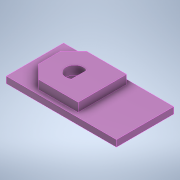
# Autodesk Inventor part: AngleSensor
Saved by Autodesk Inventor 2022 (Build 260153000, 153)
## iProperties
Created: 2021-12-29
Part Number: AngleSensor
Material: Genérico
Document SubType Name: Modeling
Designer: JK
Density: 1 g/cm^3
Appearance: Suave - Púrpura
Author: JK
Autodesk Inventor part; units mm, degrees
ref_plane "YZ Plane" through (0, 0, 0) normal (1, 0, 0) x (0, 1, 0)
ref_plane "XZ Plane" through (0, 0, 0) normal (0, 1, 0) x (-1, 0, 0)
ref_plane "XY Plane" through (0, 0, 0) normal (0, 0, 1) x (1, 0, 0)
sketch "Boceto1" plane through (0, 0, 0) normal (0, 1, 0) x (-1, 0, 0)
  line L0 (-12.5, 6.5) -> (12.5, 6.5)
  line L1 (12.5, 6.5) -> (12.5, -6.5)
  line L2 (12.5, -6.5) -> (-12.5, -6.5)
  line L3 (-12.5, -6.5) -> (-12.5, 6.5)
  line L4 (-12.5, 6.5) -> (12.5, -6.5) construction
  line L5 (12.5, 6.5) -> (-12.5, -6.5) construction
  point P0 (0, 0)
  dimension "d0" = 13
  dimension "d1" = 25
  constraints: 12 end point, 2 midpoint, 2 parallel, 1 horizontal, 1 perpendicular
  measures "d0" distance of L0.end L1.end
  measures "d1" distance of L1.end L2.end
extrude "Extrusión1" add sketch "Boceto1" along normal blind 1.5
sketch "Boceto2" plane through (0, 1.5, 0) normal (0, 1, 0) x (1, 0, 0)
  circle A0 centre (-3.5, 0) radius 2.75
  line L0 (-12.5, 6.5) -> (-12.5, -6.5) projected
  point P0 (0, 0)
  dimension "d4" = 9
  dimension "d5" = 5.5
  constraints: 1 centre point
  measures "d4" distance from line of L0 A0.centre
  measures "d5" diameter of A0
extrude "Extrusión2" cut sketch "Boceto2" against normal blind 1.5
sketch "Boceto3" plane through (0, 1.5, 0) normal (0, 1, 0) x (1, 0, 0)
  line L0 (-9.2, -5.5) -> (2.8, -5.5)
  line L1 (2.8, -5.5) -> (2.8, 5.5)
  line L2 (2.8, 5.5) -> (-9.2, 5.5)
  line L3 (-9.2, 5.5) -> (-9.2, -5.5)
  line L4 (-12.5, 6.5) -> (-12.5, -6.5) projected
  line L5 (12.5, 6.5) -> (-12.5, 6.5) projected
  circle A0 centre (-3.5, 0) radius 2.75 projected
  circle A1 centre (-3.5, 0) radius 2
  point P0 (0, 0)
  dimension "d8" = 11
  dimension "d9" = 12
  dimension "d10" = 3.3
  dimension "d11" = 1
  dimension "d14" = 4
  constraints: 8 end point, 2 parallel, 1 centre point, 1 coincident, 1 horizontal, 1 perpendicular
  measures "d8" distance between parallel lines of L2 L0
  measures "d9" distance between parallel lines of L3 L1
  measures "d10" distance between parallel lines of L4 L3
  measures "d11" distance between parallel lines of L5 L2
  measures "d14" diameter of A1
extrude "Extrusión3" add sketch "Boceto3" along normal blind 2 contours L3 L2 L1 L0 | A0
chamfer "Chaflán1" distance 3 angle 45 2 edges at (-9.2, 2.5, 5.5) (-9.2, 2.5, -5.5)
sketch "Boceto4" plane through (0, 3.5, 0) normal (0, 1, 0) x (1, 0, 0)
  circle A0 centre (-3.5, 0) radius 2 projected
  line L0 (-2.5075, -1.7363) -> (-2.5075, 1.7363)
  point P0 (0, 0)
  constraints: 2 end point, 2 point on circle, 1 vertical
extrude "Extrusión4" add sketch "Boceto4" against normal up to surface (2 mm away) contours A0 L0 picked at (-2.1717, 0)
